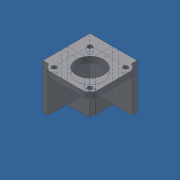
# Autodesk Inventor part: StepperXYHolder
Saved by Autodesk Inventor 2021 (Build 250183000, 183)
## iProperties
Created: 2022-08-30
Part Number: StepperXYHolder
Material: Generic
Document SubType Name: Modeling
Designer: Nathann
Density: 1 g/cm^3
Appearance: Default
Author: Nathann
Autodesk Inventor part; units mm, degrees
ref_plane "YZ Plane" through (0, 0, 0) normal (1, 0, 0) x (0, 1, 0)
ref_plane "XZ Plane" through (0, 0, 0) normal (0, 1, 0) x (-1, 0, 0)
ref_plane "XY Plane" through (0, 0, 0) normal (0, 0, 1) x (1, 0, 0)
sketch "Sketch1" plane through (0, 0, 0) normal (0, 0, 1) x (1, 0, 0)
  arc A0 (-20.5392, 17.1146) -> (-21.125, 15.7004) centre (-19.125, 15.7004) ccw projected
  line L0 (-21.125, -15.7004) -> (-21.125, 15.7004) projected
  arc A1 (-21.125, -15.7004) -> (-20.5392, -17.1146) centre (-19.125, -15.7004) ccw projected
  line L1 (-20.5392, -17.1146) -> (-17.1146, -20.5392) projected
  arc A2 (-17.1146, -20.5392) -> (-15.7004, -21.125) centre (-15.7004, -19.125) ccw projected
  line L2 (15.7004, -21.125) -> (-15.7004, -21.125) projected
  arc A3 (15.7004, -21.125) -> (17.1146, -20.5392) centre (15.7004, -19.125) ccw projected
  line L3 (20.5392, -17.1146) -> (17.1146, -20.5392) projected
  arc A4 (20.5392, -17.1146) -> (21.125, -15.7004) centre (19.125, -15.7004) ccw projected
  line L4 (21.125, 15.7004) -> (21.125, -15.7004) projected
  arc A5 (21.125, 15.7004) -> (20.5392, 17.1146) centre (19.125, 15.7004) ccw projected
  line L5 (20.5392, 17.1146) -> (17.1146, 20.5392) projected
  arc A6 (17.1146, 20.5392) -> (15.7004, 21.125) centre (15.7004, 19.125) ccw projected
  line L6 (-15.7004, 21.125) -> (15.7004, 21.125) projected
  arc A7 (-15.7004, 21.125) -> (-17.1146, 20.5392) centre (-15.7004, 19.125) ccw projected
  line L7 (-20.5392, 17.1146) -> (-17.1146, 20.5392) projected
  circle A8 centre (0, 0) radius 16 projected
  circle A9 centre (-15.875, -15.875) radius 1.625 projected
  circle A10 centre (15.875, 15.875) radius 1.625 projected
  circle A11 centre (-15.875, 15.875) radius 1.625 projected
  circle A12 centre (15.875, -15.875) radius 1.625 projected
  circle A13 centre (0, 0) radius 12
  circle A14 centre (-15.875, 15.875) radius 2
  circle A15 centre (15.875, 15.875) radius 2
  circle A16 centre (15.875, -15.875) radius 2
  circle A17 centre (-15.875, -15.875) radius 2
  point P0 (0, 0)
  dimension "d0" = 24
  dimension "d1" = 4
  dimension "d2" = 4
  dimension "d3" = 4
  dimension "d4" = 4
  constraints: 5 centre point, 4 coincident
  measures "d0" diameter of A13
  measures "d1" diameter of A14
  measures "d2" diameter of A15
  measures "d3" diameter of A16
  measures "d4" diameter of A17
extrude "Extrusion1" add sketch "Sketch1" along normal blind 5 contours L7 A7 L6 A6 L5 A5 L4 A4 L3 A3 L2 A2 L1 A1 L0 A0 | A8
sketch "Sketch3" plane through (0, 0, 5) normal (0, 0, 1) x (1, 0, 0)
  line L0 (-15.7004, 21.125) -> (15.7004, 21.125) projected
  line L1 (15.7004, 21.125) -> (-46.125, 21.125)
  line L2 (-46.125, 21.125) -> (-46.125, 26.125)
  line L3 (-46.125, 26.125) -> (15.7004, 26.125)
  line L4 (15.7004, 26.125) -> (15.7004, 21.125)
  line L5 (-21.125, 15.7004) -> (-21.125, -15.7004) projected
  line L6 (-21.125, -15.7004) -> (-26.125, -15.7004)
  line L7 (-26.125, -15.7004) -> (-26.125, 46.125)
  line L8 (-26.125, 46.125) -> (-21.125, 46.125)
  line L9 (-21.125, 46.125) -> (-21.125, -15.7004)
  point P0 (0, 0)
  dimension "d11" = 5
  dimension "d12" = 5
  dimension "d13" = 20
  dimension "d14" = 20
  constraints: 16 end point, 4 parallel, 2 horizontal, 2 perpendicular
  measures "d11" distance of L7.end L8.end
  measures "d12" distance of L1.end L2.end
  measures "d13" distance between parallel lines of L2 L7
  measures "d14" distance between parallel lines of L8 L3
extrude "Extrusion3" add sketch "Sketch3" against normal blind 40
sketch "Sketch4" plane through (0, 0, 5) normal (0, 0, 1) x (1, 0, 0)
  arc A0 (-15.7004, 21.125) -> (-17.1146, 20.5392) centre (-15.7004, 19.125) ccw projected
  line L0 (-17.1146, 20.5392) -> (-20.5392, 17.1146) projected
  arc A1 (-20.5392, 17.1146) -> (-21.125, 15.7004) centre (-19.125, 15.7004) ccw projected
  line L1 (-21.125, 21.125) -> (-21.125, 15.7004) projected
  line L2 (-15.7004, 21.125) -> (-21.125, 21.125) projected
  circle A2 centre (0, 0) radius 12 projected
  circle A3 centre (-15.875, -15.875) radius 2 projected
  circle A4 centre (15.875, -15.875) radius 2 projected
  circle A5 centre (15.875, 15.875) radius 2 projected
  circle A6 centre (-15.875, 15.875) radius 2 projected
  line L3 (15.7004, 26.125) -> (15.7004, 21.125) projected
  line L4 (-21.125, 26.125) -> (15.7004, 26.125) projected
  line L5 (-21.125, 46.125) -> (-21.125, 26.125) projected
  line L6 (-26.125, 46.125) -> (-21.125, 46.125) projected
  line L7 (-26.125, 26.125) -> (-26.125, 46.125) projected
  line L8 (-46.125, 26.125) -> (-26.125, 26.125) projected
  line L9 (-46.125, 21.125) -> (-46.125, 26.125) projected
  line L10 (-26.125, 21.125) -> (-46.125, 21.125) projected
  line L11 (-26.125, -15.7004) -> (-26.125, 21.125) projected
  line L12 (-21.125, -15.7004) -> (-26.125, -15.7004) projected
  arc A7 (-21.125, -15.7004) -> (-20.5392, -17.1146) centre (-19.125, -15.7004) ccw projected
  line L13 (-20.5392, -17.1146) -> (-17.1146, -20.5392) projected
  arc A8 (-17.1146, -20.5392) -> (-15.7004, -21.125) centre (-15.7004, -19.125) ccw projected
  line L14 (-15.7004, -21.125) -> (15.7004, -21.125) projected
  arc A9 (15.7004, -21.125) -> (17.1146, -20.5392) centre (15.7004, -19.125) ccw projected
  line L15 (17.1146, -20.5392) -> (20.5392, -17.1146) projected
  arc A10 (20.5392, -17.1146) -> (21.125, -15.7004) centre (19.125, -15.7004) ccw projected
  line L16 (21.125, -15.7004) -> (21.125, 15.7004) projected
  arc A11 (21.125, 15.7004) -> (20.5392, 17.1146) centre (19.125, 15.7004) ccw projected
  line L17 (20.5392, 17.1146) -> (17.1146, 20.5392) projected
  arc A12 (17.1146, 20.5392) -> (15.7004, 21.125) centre (15.7004, 19.125) ccw projected
  point P0 (0, 0)
extrude "Extrusion4" add sketch "Sketch4" against normal blind 5 contours A0 L0 A1 L1 L2
sketch "Sketch11" plane through (0, 0, 5) normal (0, 0, 1) x (1, 0, 0)
  line L0 (-26.125, 26.125) -> (-26.125, 46.125) projected
  line L1 (-26.125, 26.125) -> (-13.6996, 26.125)
  line L2 (-13.6996, 26.125) -> (-13.6996, 46.125)
  line L3 (-13.6996, 46.125) -> (-26.125, 46.125)
  line L4 (-26.125, 46.125) -> (-26.125, 26.125)
  line L5 (-46.125, 21.125) -> (-46.125, 26.125) projected
  line L6 (-46.125, 26.125) -> (-26.125, 26.125)
  line L7 (-26.125, 26.125) -> (-26.125, 13.3287)
  line L8 (-26.125, 13.3287) -> (-46.125, 13.3287)
  line L9 (-46.125, 13.3287) -> (-46.125, 26.125)
  point P0 (0, 0)
  constraints: 16 end point, 4 parallel, 2 horizontal, 2 perpendicular, 1 point on line
extrude "Extrusion9" cut sketch "Sketch11" against normal blind 20
sketch "Sketch7" plane through (0, 0, -35) normal (0, 0, -1) x (-1, 0, 0)
  line L0 (21.625, 21.625) -> (-23.2924, 21.625)
  line L1 (-23.2924, 21.625) -> (-23.2924, -21.9013)
  line L2 (-23.2924, -21.9013) -> (21.625, -21.9013)
  line L3 (21.625, -21.9013) -> (21.625, 21.625)
  line L4 (-15.7004, 21.125) -> (21.125, 21.125) projected
  line L5 (21.125, 21.125) -> (21.125, -15.7004) projected
  point P0 (0, 0)
  dimension "d35" = 0.5
  dimension "d36" = 0.5
  constraints: 8 end point, 2 parallel, 1 horizontal, 1 perpendicular
  measures "d35" distance between parallel lines of L4 L0
  measures "d36" distance between parallel lines of L3 L5
extrude "Extrusion7" cut sketch "Sketch7" against normal blind 35
sketch "Sketch12" plane through (0, 0, -35) normal (0, 0, -1) x (-1, 0, 0)
  line L0 (46.125, 21.125) -> (46.125, 26.125) projected
  line L1 (26.125, 26.125) -> (-15.7004, 26.125) projected
  line L2 (46.125, 21.125) -> (21.6284, 21.125)
  line L3 (21.6284, 21.125) -> (21.6284, 26.125)
  line L4 (21.6284, 26.125) -> (46.125, 26.125)
  line L5 (46.125, 26.125) -> (46.125, 21.125)
  line L6 (26.125, 46.125) -> (21.125, 46.125) projected
  line L7 (-15.7004, 21.625) -> (21.625, 21.625) projected
  line L8 (26.125, 46.125) -> (21.125, 46.125)
  line L9 (21.125, 46.125) -> (21.125, 21.625)
  line L10 (21.125, 21.625) -> (26.125, 21.625)
  line L11 (26.125, 21.625) -> (26.125, 46.125)
  point P0 (0, 0)
  point P1 (21.125, 26.125)
  dimension "d54" = 5
  dimension "d55" = 5
  dimension "d56" = 4.5
  dimension "d57" = 0.5
  constraints: 16 end point, 4 parallel, 2 horizontal, 2 perpendicular, 2 point on line
  measures "d54" distance of L9.end L10.end
  measures "d55" distance of L2.end L3.end
  measures "d56" distance between parallel lines of L1 L10
  measures "d57" distance between parallel lines of L10 L2
extrude "Extrusion10" add sketch "Sketch12" along normal blind 20 contours L2 L3 L10 L11 L4 L0 | L11 L10 L3 L1 | L1 L9 L6 L11
sketch "Sketch13" plane through (-46.125, 21.125, -15) normal (0, -1, 0) x (1, 0, 0)
  circle A0 centre (10, -30) radius 2.5
  circle A1 centre (10, -10) radius 2.5
  line L0 (24.4966, -40) -> (0, -40) projected
  line L1 (0, 0) -> (0, -40) projected
  point P0 (46.125, 15)
  dimension "d60" = 10
  dimension "d61" = 10
  dimension "d62" = 5
  dimension "d63" = 5
  dimension "d64" = 20
  dimension "d65" = 10
  constraints: 2 centre point
  measures "d60" distance from line of L0 A0.centre
  measures "d61" distance from line of L1 A0.centre
  measures "d62" diameter of A0
  measures "d63" diameter of A1
  measures "d64" distance of A0.centre A1.centre
  measures "d65" distance from line of L1 A1.centre
extrude "Extrusion11" cut sketch "Sketch13" against normal blind 20
sketch "Sketch14" plane through (-26.125, 26.125, -15) normal (-1, 0, 0) x (0, 0, 1)
  circle A0 centre (-10, 10) radius 2.5
  circle A1 centre (-30, 10) radius 2.5
  line L0 (0, 0) -> (0, 20) projected
  line L1 (0, 20) -> (-40, 20) projected
  point P0 (15, -26.125)
  dimension "d68" = 10
  dimension "d69" = 10
  dimension "d70" = 20
  dimension "d71" = 10
  dimension "d72" = 5
  dimension "d73" = 5
  constraints: 2 centre point
  measures "d68" distance from line of L0 A0.centre
  measures "d69" distance from line of L1 A0.centre
  measures "d70" distance of A0.centre A1.centre
  measures "d71" distance from line of L1 A1.centre
  measures "d72" diameter of A1
  measures "d73" diameter of A0
extrude "Extrusion12" cut sketch "Sketch14" against normal blind 20
equation "\"d36\" = d35"
body "Solid1"
